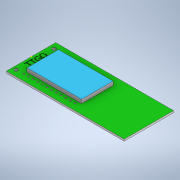
# Autodesk Inventor part: lora32Placa
Saved by Autodesk Inventor 2020 (Build 240168000, 168)
## iProperties
Created: 2021-10-19
Part Number: lora32Placa
Material: Genérico
Document SubType Name: Modeling
Designer: DANIEL
Density: 1 g/cm^3
Appearance: Valor por defecto
Author: DANIEL
Autodesk Inventor part; units mm, degrees
ref_plane "YZ Plane" through (0, 0, 0) normal (1, 0, 0) x (0, 1, 0)
ref_plane "XZ Plane" through (0, 0, 0) normal (0, 1, 0) x (-1, 0, 0)
ref_plane "XY Plane" through (0, 0, 0) normal (0, 0, 1) x (1, 0, 0)
sketch "Boceto1" plane through (0, 0, 0) normal (1, 0, 0) x (0, 1, 0)
  line L0 (0.7564, 13.5) -> (-0.2436, 13.5)
  line L1 (-0.2436, 13.5) -> (-0.2436, -13.5)
  line L2 (-0.2436, -13.5) -> (0.7564, -13.5)
  line L3 (0.7564, -13.5) -> (0.7564, 13.5)
  point P0 (0, 0)
  dimension "d0" = 1
  dimension "d1" = 27
  dimension "d2" = 13.5
  constraints: 8 end point, 2 parallel, 1 horizontal, 1 perpendicular
  measures "d0" distance between parallel lines of L1 L3
  measures "d1" distance between parallel lines of L2 L0
  measures "d2" distance from line of L2 point (0, 0)
extrude "Extrusión1" add sketch "Boceto1" along normal blind 64.47
sketch "Boceto2" plane through (0, -0.2436, -13.5) normal (0, -1, 0) x (1, 0, 0)
  line L0 (0, 0) -> (64.47, 0) projected
  line L1 (0, 27) -> (0, 0) projected
  line L2 (0, 27) -> (0, 0) projected
  line L3 (0, 0) -> (64.47, 0) projected
  line L4 (64.47, 27) -> (64.47, 0) projected
  line L5 (0, 27) -> (64.47, 27) projected
  line L6 (0, 13.5) -> (64.47, 13.5)
  line L7 (64.47, 0) -> (64.47, 27) projected
  point P0 (2.56, 3.44)
  point P1 (6.1, 3.44)
  point P2 (8.64, 3.44)
  point P3 (16.26, 3.44)
  point P4 (18.8, 3.44)
  point P5 (21.34, 3.44)
  point P6 (23.88, 3.44)
  point P7 (26.42, 3.44)
  point P8 (28.96, 3.44)
  point P9 (31.5, 3.44)
  point P10 (34.04, 3.44)
  point P11 (11.18, 3.44)
  point P12 (13.72, 3.44)
  point P13 (2.56, 23.56)
  point P14 (6.1, 23.56)
  point P15 (8.64, 23.56)
  point P16 (16.26, 23.56)
  point P17 (18.8, 23.56)
  point P18 (21.34, 23.56)
  point P19 (23.88, 23.56)
  point P20 (26.42, 23.56)
  point P21 (28.96, 23.56)
  point P22 (31.5, 23.56)
  point P23 (34.04, 23.56)
  point P24 (11.18, 23.56)
  point P25 (13.72, 23.56)
  dimension "d5" = 3.44
  dimension "d6" = 2.56
  dimension "d8" = 2.54
  dimension "d9" = 2.54
  dimension "d10" = 2.54
  dimension "d11" = 2.54
  dimension "d12" = 2.54
  dimension "d13" = 2.54
  dimension "d14" = 2.54
  dimension "d15" = 2.54
  dimension "d16" = 2.54
  dimension "d17" = 2.54
  dimension "d18" = 2.54
  dimension "d19" = 3.54
  constraints: 13 symmetric about line, 5 horizontal alignment, 2 end point, 1 midpoint
  measures "d5" distance from line of L0 point (2.56, 3.44)
  measures "d6" distance from line of L1 point (2.56, 3.44)
  measures "d8" distance of point (6.1, 3.44) point (8.64, 3.44)
  measures "d9" distance of point (8.64, 3.44) point (11.18, 3.44)
  measures "d10" distance of point (11.18, 3.44) point (13.72, 3.44)
  measures "d11" distance of point (13.72, 3.44) point (16.26, 3.44)
  measures "d12" distance of point (18.8, 3.44) point (16.26, 3.44)
  measures "d13" distance of point (18.8, 3.44) point (21.34, 3.44)
  measures "d14" distance of point (21.34, 3.44) point (23.88, 3.44)
  measures "d15" distance of point (23.88, 3.44) point (26.42, 3.44)
  measures "d16" distance of point (26.42, 3.44) point (28.96, 3.44)
  measures "d17" distance of point (28.96, 3.44) point (31.5, 3.44)
  measures "d18" distance of point (31.5, 3.44) point (34.04, 3.44)
  measures "d19" distance of point (6.1, 3.44) point (2.56, 3.44)
hole "Agujero1" at (2.56, -0.2436, -10.06) at (6.1, -0.2436, -10.06) at (8.64, -0.2436, -10.06) at (16.26, -0.2436, -10.06) at (18.8, -0.2436, -10.06) at (21.34, -0.2436, -10.06) at (23.88, -0.2436, -10.06) at (26.42, -0.2436, -10.06) at (28.96, -0.2436, -10.06) at (31.5, -0.2436, -10.06) at (34.04, -0.2436, -10.06) at (11.18, -0.2436, -10.06) at (13.72, -0.2436, -10.06) at (34.04, -0.2436, 10.06) at (31.5, -0.2436, 10.06) at (28.96, -0.2436, 10.06) at (26.42, -0.2436, 10.06) at (23.88, -0.2436, 10.06) at (21.34, -0.2436, 10.06) at (18.8, -0.2436, 10.06) at (16.26, -0.2436, 10.06) at (13.72, -0.2436, 10.06) at (11.18, -0.2436, 10.06) at (8.64, -0.2436, 10.06) at (6.1, -0.2436, 10.06) at (2.56, -0.2436, 10.06) direction (0, 1, 0) diameter 0.9 end through all
sketch "Boceto3" plane through (0, -0.2436, -13.5) normal (0, -1, 0) x (1, 0, 0)
  circle A0 centre (2.56, 3.44) radius 0.45 projected
  point P0 (0, 13.5)
  point P1 (2.1371, 23.7139)
  constraints: 1 coincident
hole "Agujero2" at (2.56, -0.2436, -10.06) at (2.1371, -0.2436, 10.2139) direction (0, 1, 0) diameter 2 end through all
sketch "Boceto4" plane through (0, -0.2436, -13.5) normal (0, -1, 0) x (1, 0, 0)
  point P0 (0, 13.5)
ref_plane "Plano de trabajo1" through (0, -0.2436, -13.5) normal (0, -1, 0) x (1, 0, 0)
ref_plane "Plano de trabajo5" through (0, -0.2436, 11.183) normal (0, 0, 1) x (1, 0, 0)
ref_plane "Plano de trabajo6" through (64.47, 0.7564, -11.183) normal (0, 0, -1) x (-1, 0, 0)
sketch "Boceto5" plane through (0, 0.7564, 13.5) normal (0, 1, 0) x (1, 0, 0)
  line L0 (1.1898, 7.974) -> (1.1898, 18.6346) construction
  line L1 (1.1898, 18.6346) -> (4.3663, 18.6346) construction
  line L2 (4.3663, 18.6346) -> (4.3663, 7.974) construction
  line L3 (4.3663, 7.974) -> (1.1898, 7.974) construction
  line L4 (6.1, 5.127) -> (36.0028, 5.127)
  line L5 (36.0028, 5.127) -> (36.0028, 22.4329)
  line L6 (36.0028, 22.4329) -> (6.1, 22.4329)
  line L7 (6.1, 22.4329) -> (6.1, 5.127)
  point P0 (0, 13.5)
  constraints: 8 end point, 2 parallel, 1 horizontal, 1 perpendicular, 2 other
extrude "Extrusión2" add sketch "Boceto5" along normal blind 2
sketch "Boceto6" plane through (0, 0.7564, 13.5) normal (0, 1, 0) x (1, 0, 0)
  line L0 (1.1904, 8.2396) -> (1.1904, 18.9001) construction
  line L1 (1.1904, 18.9001) -> (4.3668, 18.9001) construction
  line L2 (4.3668, 18.9001) -> (4.3668, 8.2396) construction
  line L3 (4.3668, 8.2396) -> (1.1904, 8.2396) construction
  point P0 (0, 13.5)
  constraints: 2 other
sketch "Boceto7" plane through (0, -0.2436, -13.5) normal (0, -1, 0) x (1, 0, 0)
  line L0 (0, 27) -> (64.47, 27) projected
  line L1 (64.47, 27) -> (64.47, 0) projected
  line L2 (62.97, 14) -> (61.97, 14)
  line L3 (61.97, 14) -> (61.97, 13)
  line L4 (61.97, 13) -> (62.97, 13)
  line L5 (62.97, 13) -> (62.97, 14)
  point P0 (0, 13.5)
  point P1 (62.47, 13.5)
  dimension "d43" = 13.5
  dimension "d44" = 2
  dimension "d45" = 1
  dimension "d46" = 1
  dimension "d47" = 0.5
  dimension "d48" = 0.5
  constraints: 8 end point, 2 parallel, 1 horizontal, 1 perpendicular
  measures "d43" distance from line of L0 point (62.47, 13.5)
  measures "d44" distance from line of point (62.47, 13.5) L1
  measures "d45" distance between parallel lines of L3 L5
  measures "d46" distance between parallel lines of L4 L2
  measures "d47" distance from line of L2 point (62.47, 13.5)
  measures "d48" distance from line of L3 point (62.47, 13.5)
extrude "Extrusión3" add sketch "Boceto7" along normal blind 0.2
equation "\"d8\" = L"
equation "\"d9\" = L"
equation "\"d10\" = L"
equation "\"d11\" = L"
equation "\"d12\" = L"
equation "\"d13\" = L"
equation "\"d14\" = L"
equation "\"d15\" = L"
equation "\"d16\" = L"
equation "\"d17\" = L"
equation "\"d18\" = L"
equation "\"L\" = 2.54"
